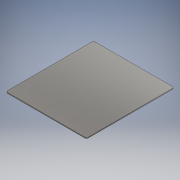
# Autodesk Inventor part: BatteryPlate
Saved by Autodesk Inventor 2018 (Build 220112000, 112)
## iProperties
Created: 2017-11-21
Part Number: BatteryPlate
Material: Steel, Galvanized
Document SubType Name: Modeling
Designer: P136265
Density: 7.85 g/cm^3
Appearance: Galvanized
Author: P136265
Autodesk Inventor part; units mm, degrees
ref_plane "YZ Plane" through (0, 0, 0) normal (1, 0, 0) x (0, 1, 0)
ref_plane "XZ Plane" through (0, 0, 0) normal (0, 1, 0) x (-1, 0, 0)
ref_plane "XY Plane" through (0, 0, 0) normal (0, 0, 1) x (1, 0, 0)
sketch "Sketch1" plane through (0, 0, 0) normal (0, 0, 1) x (1, 0, 0)
  line L0 (-110, 125) -> (110, 125)
  line L1 (115, 120) -> (115, -120)
  line L2 (110, -125) -> (-110, -125)
  line L3 (-115, -120) -> (-115, 120)
  line L4 (-115, 125) -> (115, -125) construction
  line L5 (115, 125) -> (-115, -125) construction
  arc A0 (-110, 125) -> (-115, 120) centre (-110, 120) ccw
  arc A1 (115, 120) -> (110, 125) centre (110, 120) ccw
  arc A2 (110, -125) -> (115, -120) centre (110, -120) ccw
  arc A3 (-115, -120) -> (-110, -125) centre (-110, -120) ccw
  point P0 (0, 0)
  dimension "d0" = 230
  dimension "d1" = 250
  dimension "d2" = 5
  constraints: 12 end point, 8 point on circle, 8 point on line, 8 tangent, 4 centre point, 3 equal radius, 2 midpoint, 2 parallel, 1 horizontal, 1 perpendicular
  measures "d0" distance of L4.end L5.end
  measures "d1" distance of L5.start L4.end
  measures "d2" radius of A0
extrude "Extrusion1" add sketch "Sketch1" along normal blind 2.5
body "Solid1"
